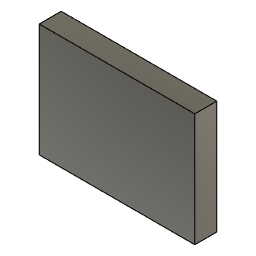
Assembled v4 (Autodesk Fusion 360 archive; units mm, degrees)
design "Temperature Sensor"
Autodesk Fusion 360 part; units mm, degrees
sketch "Sketch1" plane through (0, 0, 0) normal (0, 0, 1) x (1, 0, 0)
  line L0 (0, 0) -> (35, 0)
  line L1 (35, 0) -> (35, 4.95)
  line L2 (35, 4.95) -> (0, 4.95)
  line L3 (0, 4.95) -> (0, 0)
  dimension "d1" = 35
  dimension "d2" = 4.95
  constraint horizontal L0
  constraint vertical L1
  constraint horizontal L2
  constraint vertical L3
  constraint coincident L0.start L3.end
  measures "d1" distance of L0.start L0.end
  measures "d2" distance of L0.start L2.end
extrude "Extrude1" add sketch "Sketch1" along normal blind 25.5

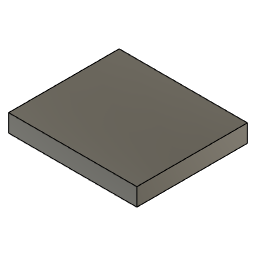
design "Transciever"
Autodesk Fusion 360 part; units mm, degrees
sketch "Sketch1" plane through (0, 0, 0) normal (0, 0, 1) x (1, 0, 0)
  line L0 (0, 0) -> (29, 0)
  line L1 (29, 0) -> (29, 25)
  line L2 (29, 25) -> (0, 25)
  line L3 (0, 25) -> (0, 0)
  dimension "d1" = 25
  dimension "d2" = 29
  constraint horizontal L0
  constraint vertical L1
  constraint horizontal L2
  constraint vertical L3
  constraint coincident L0.start L3.end
  measures "d1" distance of L0.start L2.end
  measures "d2" distance of L0.start L0.end
extrude "Extrude1" add sketch "Sketch1" along normal blind 4

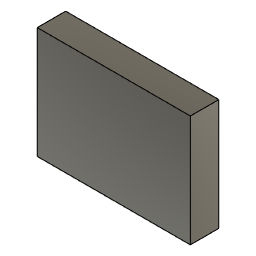
design "GPS"
Autodesk Fusion 360 part; units mm, degrees
sketch "Sketch1" plane through (0, 0, 0) normal (0, 0, 1) x (1, 0, 0)
  line L0 (0, 0) -> (35, 0)
  line L1 (35, 0) -> (35, 6.5)
  line L2 (35, 6.5) -> (0, 6.5)
  line L3 (0, 6.5) -> (0, 0)
  dimension "d1" = 35
  dimension "d2" = 6.5
  constraint horizontal L0
  constraint vertical L1
  constraint horizontal L2
  constraint vertical L3
  constraint coincident L0.start L3.end
  measures "d1" distance of L0.start L0.end
  measures "d2" distance of L0.start L2.end
extrude "Extrude1" add sketch "Sketch1" along normal blind 25.5

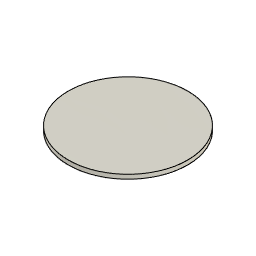
design "Top Top"
Autodesk Fusion 360 part; units mm, degrees
sketch "Sketch1" plane through (0, 0, 0) normal (0, 0, 1) x (1, 0, 0)
  circle A0 centre (0, 0) radius 28
  dimension "d1" = 56
  constraint coincident A0.centre origin
  measures "d1" diameter of A0
extrude "Extrude1" add sketch "Sketch1" along normal blind 2

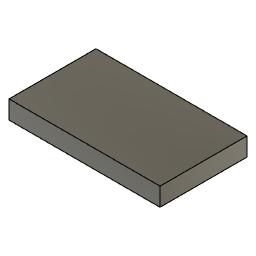
design "Accelerometer"
Autodesk Fusion 360 part; units mm, degrees
sketch "Sketch1" plane through (0, 0, 0) normal (0, 0, 1) x (1, 0, 0)
  line L0 (0, 0) -> (13.2, 0)
  line L1 (13.2, 0) -> (13.2, 7.6)
  line L2 (13.2, 7.6) -> (0, 7.6)
  line L3 (0, 7.6) -> (0, 0)
  dimension "d1" = 13.2
  dimension "d2" = 7.6
  constraint horizontal L0
  constraint vertical L1
  constraint horizontal L2
  constraint vertical L3
  constraint coincident L0.start L3.end
  measures "d1" distance of L0.start L0.end
  measures "d2" distance of L0.start L2.end
extrude "Extrude1" add sketch "Sketch1" along normal blind 1.6

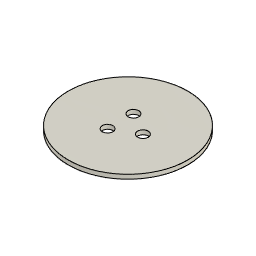
design "Top Lid"
Autodesk Fusion 360 part; units mm, degrees
sketch "Sketch1" plane through (0, 0, 0) normal (0, 0, 1) x (1, 0, 0)
  circle A0 centre (0, 0) radius 28
  dimension "d1" = 56
  constraint coincident A0.centre origin
  measures "d1" diameter of A0
extrude "Extrude1" add sketch "Sketch1" along normal blind 2
sketch "Sketch2" plane through (0, 0, 2) normal (0, 0, 1) x (-1, 0, 0)
  circle A0 centre (0, 0) radius 28
  circle A1 centre (-7, 0) radius 2.5
  dimension "d5" = 5
  measures "d5" diameter of A1
extrude "Extrude2" cut sketch "Sketch2" against normal blind 10 contours A1
pattern_circular "C-Pattern1" count 3 over 360 about axis through (0, 0, 1.75) along (0, 0, 1) of 1 faces at (4.5124, 0.2489, 0.6667)

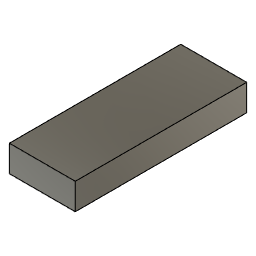
design "ArduinoZeroMKR"
Autodesk Fusion 360 part; units mm, degrees
sketch "Sketch1" plane through (0, 0, 0) normal (0, 0, 1) x (1, 0, 0)
  line L0 (0, 0) -> (25, 0)
  line L1 (25, 0) -> (25, 65)
  line L2 (25, 65) -> (0, 65)
  line L3 (0, 65) -> (0, 0)
  dimension "d1" = 25
  dimension "d2" = 65
  constraint horizontal L0
  constraint vertical L1
  constraint horizontal L2
  constraint vertical L3
  constraint coincident L0.start L3.end
  measures "d1" distance of L0.start L0.end
  measures "d2" distance of L0.start L2.end
extrude "Extrude1" add sketch "Sketch1" along normal blind 10

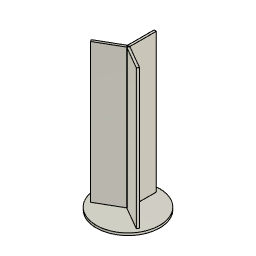
design "BottomLid"
Autodesk Fusion 360 part; units mm, degrees
sketch "Sketch1" plane through (0, 0, 0) normal (0, 0, 1) x (1, 0, 0)
  circle A0 centre (0, 0) radius 28
  dimension "d1" = 56
  constraint coincident A0.centre origin
  measures "d1" diameter of A0
extrude "Extrude1" add sketch "Sketch1" along normal blind 2 makes body 1
sketch "Sketch2" plane through (0, 0, 2) normal (0, 0, 1) x (-1, 0, 0)
  circle A0 centre (0, 0) radius 28
  line L0 (-1, 0) -> (1, 0)
  line L1 (1, 0) -> (1, -24)
  line L2 (1, -24) -> (-1, -24)
  line L3 (-1, -24) -> (-1, 0)
  line L4 (21.2846, 11.134) -> (0.5, -0.866)
  line L5 (20.2846, 12.866) -> (21.2846, 11.134)
  line L6 (-0.5, 0.866) -> (20.2846, 12.866)
  line L7 (0.5, -0.866) -> (-0.5, 0.866)
  line L8 (-20.2846, 12.866) -> (0.5, 0.866)
  line L9 (-21.2846, 11.134) -> (-20.2846, 12.866)
  line L10 (-0.5, -0.866) -> (-21.2846, 11.134)
  line L11 (0.5, 0.866) -> (-0.5, -0.866)
  dimension "d7" = 360
  constraint horizontal L0
  constraint vertical L1
  constraint horizontal L2
  constraint vertical L3
extrude "Extrude2" add sketch "Sketch2" along normal blind 123 separate body contours L0 L3 L6 L7 L8 L9 L10 | L0 L1 L4 L5 L6 L8 L11 | L1 L2 L3 L4 L7 L10 L11 makes body 2

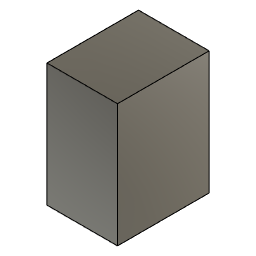
design "Barometer"
Autodesk Fusion 360 part; units mm, degrees
sketch "Sketch1" plane through (0, 0, 0) normal (0, 0, 1) x (1, 0, 0)
  line L0 (0, 0) -> (4.7, 0)
  line L1 (4.7, 0) -> (4.7, 6.1)
  line L2 (4.7, 6.1) -> (0, 6.1)
  line L3 (0, 6.1) -> (0, 0)
  dimension "d1" = 4.7
  dimension "d2" = 6.1
  constraint horizontal L0
  constraint vertical L1
  constraint horizontal L2
  constraint vertical L3
  constraint coincident L0.start L3.end
  measures "d1" distance of L0.start L0.end
  measures "d2" distance of L0.start L2.end
extrude "Extrude1" add sketch "Sketch1" along normal blind 8.2

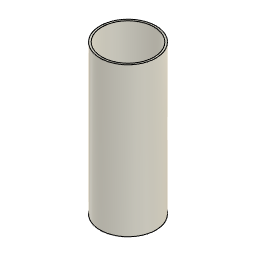
design "Main Body"
Autodesk Fusion 360 part; units mm, degrees
sketch "Sketch1" plane through (0, 0, 0) normal (1, 0, 0) x (0, 1, 0)
  line L0 (30, 0) -> (30, 160)
  line L1 (30, 160) -> (28, 160)
  line L2 (28, 160) -> (28, 0)
  line L3 (28, 0) -> (30, 0)
  dimension "d1" = 30
  dimension "d2" = 160
  dimension "d3" = 2
  constraint horizontal L1
  measures "d1" distance of origin L0.start
  measures "d2" distance of L0.start L0.end
  measures "d3" distance of L0.end L1.end
revolve "Revolve1" add sketch "Sketch1" angle 360 about axis through (0, 0, 1.75) along (0, 0, 1)
